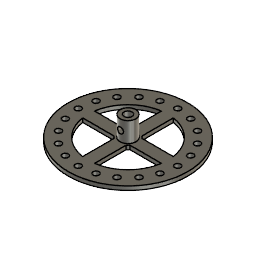
フライホイール v1 (Autodesk Fusion 360 design; units mm, degrees)
Autodesk Fusion 360 part; units mm, degrees
sketch "スケッチ1" plane through (0, 0, 0) normal (0, 0, 1) x (1, 0, 0)
  circle A0 centre (0, 0) radius 30
  circle A1 centre (0, 0) radius 20
  circle A2 centre (0, 0) radius 5
  circle A3 centre (0, 25) radius 1.5
  line L0 (-3, 4) -> (-3, 19.7737)
  line L1 (3, 4) -> (3, 19.7737)
  line L2 (-4, 3) -> (-19.7737, 3)
  line L3 (-4, -3) -> (-19.7737, -3)
  line L4 (-3, -4) -> (-3, -19.7737)
  line L5 (3, -4) -> (3, -19.7737)
  line L6 (4, -3) -> (19.7737, -3)
  line L7 (4, 3) -> (19.7737, 3)
  circle A4 centre (-7.7254, 23.7764) radius 1.5
  circle A5 centre (-14.6946, 20.2254) radius 1.5
  circle A6 centre (-20.2254, 14.6946) radius 1.5
  circle A7 centre (-23.7764, 7.7254) radius 1.5
  circle A8 centre (-25, 0) radius 1.5
  circle A9 centre (-23.7764, -7.7254) radius 1.5
  circle A10 centre (-20.2254, -14.6946) radius 1.5
  circle A11 centre (-14.6946, -20.2254) radius 1.5
  circle A12 centre (-7.7254, -23.7764) radius 1.5
  circle A13 centre (0, -25) radius 1.5
  circle A14 centre (7.7254, -23.7764) radius 1.5
  circle A15 centre (14.6946, -20.2254) radius 1.5
  circle A16 centre (20.2254, -14.6946) radius 1.5
  circle A17 centre (23.7764, -7.7254) radius 1.5
  circle A18 centre (25, 0) radius 1.5
  circle A19 centre (23.7764, 7.7254) radius 1.5
  circle A20 centre (20.2254, 14.6946) radius 1.5
  circle A21 centre (14.6946, 20.2254) radius 1.5
  circle A22 centre (7.7254, 23.7764) radius 1.5
  dimension "d2" = 360
  dimension "d4" = 360
  constraint coincident A0.centre A1.centre
  constraint concentric A0 A1
  constraint coincident A2 L0.start
  constraint coincident A1 L0.end
  constraint vertical L0
  constraint coincident A2 L1.start
  constraint coincident A1 L1.end
  constraint parallel L0 L1
extrude "押し出し1" add sketch "スケッチ1" along normal blind 2 contours A0 | A1 A2 L6 L7 | A1 A2 L0 L1 | A2 | A1 A2 L4 L5 | A1 A2 L2 L3
sketch "スケッチ2" plane through (0, 0, 2) normal (0, 0, 1) x (-1, 0, 0)
  circle A0 centre (0, -25) radius 1.5
  circle A1 centre (7.7254, 23.7764) radius 1.5
  circle A2 centre (14.6946, -20.2254) radius 1.5
  circle A3 centre (23.7764, -7.7254) radius 1.5
  circle A4 centre (14.6946, 20.2254) radius 1.5
  circle A5 centre (25, 0) radius 1.5
  circle A6 centre (20.2254, 14.6946) radius 1.5
  circle A7 centre (-7.7254, -23.7764) radius 1.5
  circle A8 centre (0, 0) radius 30
  arc A9 (-4, -3) -> (-3, -4) centre (0, 0) ccw
  line L0 (-3, -4) -> (-3, -19.7737)
  arc A10 (-19.7737, -3) -> (-3, -19.7737) centre (0, 0) ccw
  line L1 (-19.7737, -3) -> (-4, -3)
  line L2 (-3, 19.7737) -> (-3, 4)
  arc A11 (-3, 4) -> (-4, 3) centre (0, 0) ccw
  line L3 (-4, 3) -> (-19.7737, 3)
  arc A12 (-3, 19.7737) -> (-19.7737, 3) centre (0, 0) ccw
  circle A13 centre (-14.6946, 20.2254) radius 1.5
  circle A14 centre (-23.7764, -7.7254) radius 1.5
  line L4 (3, -19.7737) -> (3, -4)
  arc A15 (3, -4) -> (4, -3) centre (0, 0) ccw
  line L5 (4, -3) -> (19.7737, -3)
  arc A16 (3, -19.7737) -> (19.7737, -3) centre (0, 0) ccw
  line L6 (19.7737, 3) -> (4, 3)
  arc A17 (4, 3) -> (3, 4) centre (0, 0) ccw
  line L7 (3, 4) -> (3, 19.7737)
  arc A18 (19.7737, 3) -> (3, 19.7737) centre (0, 0) ccw
  circle A19 centre (-25, 0) radius 1.5
  circle A20 centre (-23.7764, 7.7254) radius 1.5
  circle A21 centre (23.7764, 7.7254) radius 1.5
  circle A22 centre (-14.6946, -20.2254) radius 1.5
  circle A23 centre (-20.2254, -14.6946) radius 1.5
  circle A24 centre (7.7254, -23.7764) radius 1.5
  circle A25 centre (-20.2254, 14.6946) radius 1.5
  circle A26 centre (0, 25) radius 1.5
  circle A27 centre (-7.7254, 23.7764) radius 1.5
  circle A28 centre (20.2254, -14.6946) radius 1.5
  circle A29 centre (0, 0) radius 2
  circle A30 centre (0, 0) radius 4
  constraint coincident A8.centre A9.centre
  constraint concentric A8 A30
extrude "押し出し2" add sketch "スケッチ2" along normal blind 6 contours A30
extrude "押し出し3" cut 1 faces at (-0.4157, -0.5212, 2) along direction (0, 0, -1) blind 2
extrude "押し出し4" add 1 faces at (-3.311, 0.2981, 8) along direction (0, 0, 1) blind 4
ref_plane "作業平面1" through (0, 0, 6) normal (0, 1, 0) x (0, 0, 1)
sketch "スケッチ3" plane through (0, 0, 0) normal (0, 1, 0) x (1, 0, 0)
  circle A0 centre (0, -7) radius 1.5
extrude "押し出し5" cut sketch "スケッチ3" along normal blind 4 and the other way blind 4
